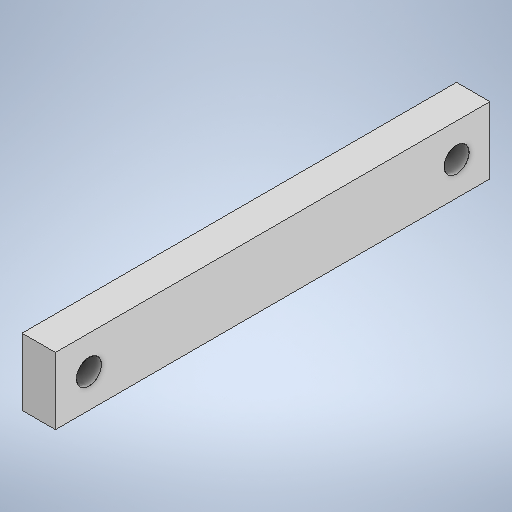
# Autodesk Inventor part: Weight Baby
Saved by Autodesk Inventor 2025 (Build 290162000, 162)
## iProperties
Created: 2024-11-22
Part Number: Weight Baby
Material: Generic
Document SubType Name: Modeling
Designer: liaco
Density: 1 g/cm^3
Appearance: Default
Author: liaco
Autodesk Inventor part; units mm, degrees
ref_plane "YZ Plane" through (0, 0, 0) normal (1, 0, 0) x (0, 1, 0)
ref_plane "XZ Plane" through (0, 0, 0) normal (0, 1, 0) x (-1, 0, 0)
ref_plane "XY Plane" through (0, 0, 0) normal (0, 0, 1) x (1, 0, 0)
sketch "Sketch1" plane through (0, 0, 0) normal (1, 0, 0) x (0, 1, 0)
  line L0 (21.8571, 39) -> (9.8571, 39)
  line L1 (9.8571, 39) -> (9.8571, -39)
  line L2 (9.8571, -39) -> (21.8571, -39)
  line L3 (21.8571, -39) -> (21.8571, 39)
  line L4 (9.8571, 0) -> (21.8571, 0)
  point P0 (0, 0)
  point P1 (15.8571, 33)
  point P2 (15.8571, -33)
  dimension "d0" = 78
  dimension "d1" = 12
  dimension "d2" = 6
  dimension "d3" = 6
  dimension "d4" = 39
  constraints: 10 end point, 2 midpoint, 2 parallel, 1 horizontal, 1 perpendicular, 1 symmetric about line
  measures "d0" distance of L2.end L0.start
  measures "d1" distance of L1.end L2.end
  measures "d2" distance from line of L0 point (15.857, 33)
  measures "d3" distance from line of L3 point (15.857, 33)
  measures "d4" distance from line of point (0, 0) L0
extrude "Extrusion1" add sketch "Sketch1" along normal blind 6
hole "Hole1" at (0, 15.8571, 33) at (0, 15.8571, -33) direction (1, 0, 0) diameter 4.5 end through all clearance for "Flat Head Machine Screw" size "M4" standard "Ansi Metric M Profile"
body "Solid1"
